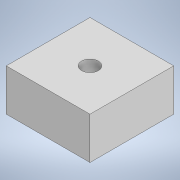
# Autodesk Inventor part: Insert Test 4mm
Saved by Autodesk Inventor 2021 (Build 250183000, 183)
## iProperties
Created: 2020-09-11
Part Number: Insert Test 4mm
Material: Generic
Document SubType Name: Modeling
Designer: cmzgt
Density: 1 g/cm^3
Appearance: Default
Author: cmzgt
Autodesk Inventor part; units mm, degrees
ref_plane "YZ Plane" through (0, 0, 0) normal (1, 0, 0) x (0, 1, 0)
ref_plane "XZ Plane" through (0, 0, 0) normal (0, 1, 0) x (-1, 0, 0)
ref_plane "XY Plane" through (0, 0, 0) normal (0, 0, 1) x (1, 0, 0)
sketch "Sketch1" plane through (0, 0, 0) normal (0, 1, 0) x (-1, 0, 0)
  line L0 (0, 0) -> (20, 0)
  line L1 (20, 0) -> (20, 20)
  line L2 (20, 20) -> (0, 20)
  line L3 (0, 20) -> (0, 0)
  dimension "d0" = 20
  dimension "d1" = 20
  constraints: 8 end point, 2 parallel, 1 horizontal, 1 perpendicular
  measures "d0" distance of L2.end L1.end
  measures "d1" distance of L1.end L0.end
extrude "Extrusion1" add sketch "Sketch1" along normal blind 10
sketch "Sketch2" plane through (0, 10, 0) normal (0, 1, 0) x (1, 0, 0)
  line L0 (0, 0) -> (-20, 0) construction
  line L1 (-10, 0) -> (-10, -20) construction
  line L2 (-20, -20) -> (0, -20) construction
  line L3 (-20, 0) -> (-20, -20) construction
  line L4 (-20, -10) -> (0, -10) construction
  line L5 (0, -20) -> (0, 0) construction
  circle A0 centre (-10, -10) radius 2
  dimension "d4" = 4
  constraints: 5 midpoint, 4 end point, 1 centre point
  measures "d4" diameter of A0
extrude "Extrusion3" cut sketch "Sketch2" against normal blind 20
body "Solid1"
